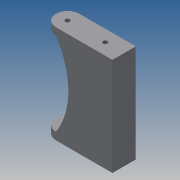
# Autodesk Inventor part: FRONT
Saved by Autodesk Inventor 2013 (Build 170138000, 138)
## iProperties
Created: 2017-02-24
Part Number: FRONT
Material: Generic
Document SubType Name: Modeling
Designer: employee
Density: 1 g/cm^3
Author: employee
Autodesk Inventor part; units mm, degrees
ref_plane "YZ Plane" through (0, 0, 0) normal (1, 0, 0) x (0, 1, 0)
ref_plane "XZ Plane" through (0, 0, 0) normal (0, 1, 0) x (-1, 0, 0)
ref_plane "XY Plane" through (0, 0, 0) normal (0, 0, 1) x (1, 0, 0)
sketch "Sketch1" plane through (0, 0, 0) normal (0, 0, 1) x (1, 0, 0)
  circle A0 centre (0, 0) radius 3
  circle A1 centre (50, 0) radius 3
  line L0 (0, 15.5) -> (65, 15.5)
  line L1 (65, 15.5) -> (65, -15.5)
  line L2 (65, -15.5) -> (0, -15.5)
  arc A2 (0, 15.5) -> (0, -15.5) centre (0, 0) ccw
  dimension "d0" = 6
  dimension "d2" = 50
  dimension "d3" = 15
  dimension "d4" = 31
  constraints: 6 end point, 3 centre point, 2 coincident, 2 point on circle, 2 tangent, 1 equal radius, 1 horizontal, 1 horizontal alignment, 1 parallel, 1 perpendicular
  measures "d0" diameter of A1
  measures "d2" distance of A1.centre point (0, 0)
  measures "d3" distance from line of L1 A1.centre
  measures "d4" distance of L0.end L1.end
extrude "Extrusion1" add sketch "Sketch1" along normal blind 10
sketch "Sketch2" plane through (65, -15.5, 0) normal (1, 0, 0) x (0, 0, -1)
  line L0 (-10, 0) -> (120, 0)
  line L1 (120, 0) -> (120, 31)
  line L2 (120, 31) -> (-10, 31)
  line L3 (-10, 31) -> (-10, 0)
  point P0 (0, 15.5)
  dimension "d7" = 130
  constraints: 8 end point, 2 parallel, 1 horizontal, 1 perpendicular
  measures "d7" distance of L1.end L2.end
extrude "Extrusion2" add sketch "Sketch2" along normal blind 10
pattern_linear "Rectangular Pattern1" count 2 spacing 120 along (0, 0, -1) of "Extrusion1"
sketch "Sketch3" plane through (0, 15.5, 10) normal (0, 1, 0) x (1, 0, 0)
  line L0 (0, 10) -> (65, 10) projected
  line L1 (65, 120) -> (0, 120) projected
  line L2 (65, 120) -> (65, 10) projected
  arc A0 (0, 10) -> (0, 120) centre (-83.5165, 65) ccw
  dimension "d13" = 100
  constraints: 2 point on circle, 1 centre point
  measures "d13" radius of A0
extrude "Extrusion3" add sketch "Sketch3" against normal blind 2
mirror "Mirror1" about plane through (0, 0, 0) normal (0, 1, 0) of "Extrusion3"
body "Solid1"
